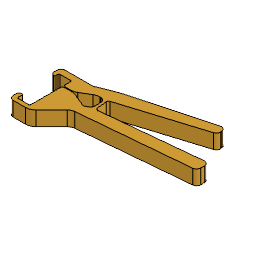
IOMOD-Puller (Autodesk Fusion 360 design; units mm, degrees)
Autodesk Fusion 360 part; units mm, degrees
note: some values were not read from the file. Set by a fixed rule: which sketch regions a step uses.
sketch "Sketch1" plane through (0, 0, 0) normal (0, 0, 1) x (1, 0, 0)
  line L0 (0, 5) -> (0, 2)
  line L1 (2, 0) -> (7.9289, 0)
  line L2 (11.4645, 1.4645) -> (18.976, 8.976)
  line L3 (21.4423, 10.1311) -> (73.1811, 14.8346)
  line L4 (75, 16.8264) -> (75, 18.7388)
  line L5 (72.7984, 20.7286) -> (26.4956, 16.038)
  line L6 (25.3999, 16.9322) -> (24.9151, 21.7179)
  line L7 (25.613, 22.7735) -> (63.4248, 34.5346)
  line L8 (64.8206, 36.6459) -> (64.76, 37.2443)
  line L9 (62.2441, 38.9723) -> (24.75, 28.75)
  line L10 (24.75, 28.75) -> (15.8665, 25.3333)
  line L11 (14.0716, 25) -> (2, 25)
  line L12 (0, 23) -> (0, 20.0001)
  line L13 (0, 20.0001) -> (1.5, 20.0001)
  line L14 (2, 20.5001) -> (2, 21.5)
  line L15 (2.5, 22) -> (7.5, 22)
  line L16 (8, 21.5) -> (8, 19)
  line L17 (9, 18) -> (11.6173, 18)
  line L18 (14.1909, 18.7132) -> (18.7957, 21.4777)
  line L19 (21.3693, 22.1909) -> (21.8547, 22.1909)
  line L20 (23.8445, 20.3925) -> (23.8704, 20.1372)
  line L21 (23.8704, 20.1372) -> (23.9618, 17.2187)
  line L22 (22.9342, 15.4078) -> (22.008, 14.8932)
  line L23 (8, 6.5218) -> (8, 2.5)
  line L24 (7.5, 2) -> (2.5, 2)
  line L25 (2, 2.5) -> (2, 4.5)
  line L26 (1.5, 5) -> (0, 5)
  arc A0 (23.8445, 20.3925) -> (21.8547, 22.1909) centre (21.8547, 20.1909) ccw
  arc A1 (73.1811, 14.8346) -> (75, 16.8264) centre (73, 16.8264) ccw
  arc A2 (75, 18.7388) -> (72.7984, 20.7286) centre (73, 18.7388) ccw
  arc A3 (63.4248, 34.5346) -> (64.8206, 36.6459) centre (62.8308, 36.4443) ccw
  arc A4 (64.76, 37.2443) -> (62.2441, 38.9723) centre (62.7702, 37.0427) ccw
  arc A5 (21.4423, 10.1311) -> (18.976, 8.976) centre (21.8044, 6.1475) ccw
  arc A6 (14.0716, 25) -> (15.8665, 25.3333) centre (14.0716, 30) ccw
  arc A7 (11.6173, 18) -> (14.1909, 18.7132) centre (11.6173, 23) ccw
  arc A8 (7.9289, 0) -> (11.4645, 1.4645) centre (7.9289, 5) ccw
  arc A9 (2, 25) -> (0, 23) centre (2, 23) ccw
  arc A10 (0, 2) -> (2, 0) centre (2, 2) ccw
  arc A11 (25.3999, 16.9322) -> (26.4956, 16.038) centre (26.3948, 17.0329) ccw
  arc A12 (25.613, 22.7735) -> (24.9151, 21.7179) centre (25.91, 21.8186) ccw
  arc A13 (21.3693, 22.1909) -> (18.7957, 21.4777) centre (21.3693, 17.1909) ccw
  arc A14 (8, 19) -> (9, 18) centre (9, 19) ccw
  arc A15 (8, 6.5247) -> (8, 6.5218) centre (9, 6.5218) ccw
  arc A16 (8, 21.5) -> (7.5, 22) centre (7.5, 21.5) ccw
  arc A17 (2.5, 22) -> (2, 21.5) centre (2.5, 21.5) ccw
  arc A18 (7.5, 2) -> (8, 2.5) centre (7.5, 2.5) ccw
  arc A19 (2, 2.5) -> (2.5, 2) centre (2.5, 2.5) ccw
  arc A20 (2, 4.5) -> (1.5, 5) centre (1.5, 4.5) ccw
  arc A21 (1.5, 20.0001) -> (2, 20.5001) centre (1.5, 20.5001) ccw
  line L27 (1, 5) -> (0, 4)
  line L28 (0.9999, 20.0001) -> (0, 21)
  arc A22 (22.9342, 15.4078) -> (23.9618, 17.2187) centre (21.9628, 17.1561) ccw
  line L29 (20.2644, 14.7966) -> (14.3954, 17.2531)
  line L30 (12.4649, 17.6408) -> (9.0149, 17.6408)
  line L31 (8.0149, 16.6422) -> (8, 6.5218)
  arc A23 (9.0149, 17.6408) -> (8.0149, 16.6422) centre (9.0149, 16.6408) ccw
  arc A24 (14.3954, 17.2531) -> (12.4649, 17.6408) centre (12.4649, 12.6408) ccw
  arc A25 (20.2644, 14.7966) -> (22.008, 14.8932) centre (21.0366, 16.6415) ccw
  point P0 (2, 5)
  dimension "d1" = 5
  dimension "d2" = 2
  dimension "d3" = 6
  dimension "d4" = 20
  dimension "d5" = 2
  dimension "d6" = 2
  dimension "d7" = 2
  dimension "d8" = 2
  dimension "d9" = 2
  dimension "d10" = 4
  dimension "d11" = 5
  dimension "d12" = 5
  dimension "d13" = 2
  dimension "d14" = 2
  dimension "d15" = 1
  dimension "d16" = 1
  dimension "d17" = 5
  dimension "d18" = 1
  dimension "d20" = 0.5
  dimension "d21" = 0.5
  dimension "d22" = 0.5
  dimension "d23" = 0.5
  dimension "d24" = 0.5
  dimension "d25" = 0.5
  dimension "d28" = 2
  dimension "d29" = 1
  dimension "d30" = 5
  dimension "d31" = 2
  constraint vertical L0
  constraint perpendicular L0 L1
  constraint perpendicular L1 L4
  constraint perpendicular L5 L6
  constraint perpendicular L5 L8
  constraint horizontal L11
  constraint perpendicular L11 L12
  constraint perpendicular L12 L13
  constraint perpendicular L13 L14
  constraint perpendicular L14 L15
  constraint perpendicular L15 L16
  constraint perpendicular L16 L17
  constraint parallel L17 L19
  constraint parallel L6 L20
  constraint vertical L23
  constraint perpendicular L23 L24
  constraint perpendicular L24 L25
  constraint perpendicular L0 L26
  constraint collinear L14 L25
  constraint collinear L16 L23
  constraint tangent L19 A0
  constraint tangent L20 A0
  constraint tangent L3 A1
  constraint tangent L4 A1
  constraint equal A0 A1
  constraint tangent L4 A2
  constraint tangent L5 A2
  constraint tangent L7 A3
  constraint tangent L8 A3
  constraint tangent L8 A4
  constraint tangent L9 A4
  constraint tangent L2 A5
  constraint tangent L3 A5
  constraint tangent L10 A6
  constraint tangent L11 A6
  constraint tangent L17 A7
  constraint tangent L18 A7
  constraint tangent L1 A8
  constraint tangent L2 A8
  constraint equal A7 A8
  constraint tangent L11 A9
  constraint tangent L12 A9
  constraint tangent L0 A10
  constraint tangent L1 A10
  constraint tangent L5 A11
  constraint tangent L6 A11
  constraint tangent L6 A12
  constraint tangent L7 A12
  constraint tangent L18 A13
  constraint tangent L19 A13
  constraint tangent L16 A14
  constraint tangent L17 A14
  constraint tangent L22 A15
  constraint tangent L23 A15
  constraint tangent L15 A16
  constraint tangent L16 A16
  constraint tangent L14 A17
  constraint tangent L15 A17
  constraint tangent L23 A18
  constraint tangent L24 A18
  constraint tangent L24 A19
  constraint tangent L25 A19
  constraint coincident P0 L25
  constraint coincident P0 L26
  constraint tangent L25 A20
  constraint tangent L26 A20
  constraint tangent L13 A21
  constraint tangent L14 A21
  constraint coincident L26 L27.start
  constraint coincident L0 L27.end
  constraint coincident L13 L28.start
  constraint coincident L12 L28.end
  constraint perpendicular L27 L28
  constraint tangent L21 A22
  constraint tangent L22 A22
  constraint parallel L11 L30
  constraint tangent L30 A23
  constraint tangent L31 A23
  constraint tangent L29 A24
  constraint tangent L30 A24
  constraint coincident L31 A15.start
  constraint tangent L29 A25
  constraint tangent L22 A25
  measures "d1" distance of L1 L26
  measures "d2" distance of L0.start P0
  measures "d3" distance of L23 L25
  measures "d4" distance of L15 L24
  measures "d5" distance of L1 L24
  measures "d6" radius of A0
  measures "d7" radius of A2
  measures "d8" radius of A3
  measures "d9" radius of A4
  measures "d10" radius of A5
  measures "d11" radius of A6
  measures "d12" radius of A7
  measures "d13" radius of A9
  measures "d14" radius of A10
  measures "d15" radius of A11
  measures "d16" radius of A12
  measures "d17" radius of A13
  measures "d18" radius of A14
  measures "d20" radius of A16
  measures "d21" radius of A17
  measures "d22" radius of A18
  measures "d23" radius of A19
  measures "d24" radius of A20
  measures "d25" radius of A21
  measures "d28" radius of A22
  measures "d29" radius of A23
  measures "d30" radius of A24
  measures "d31" radius of A25
extrude "Extrude1" add sketch "Sketch1" along normal blind 7 contours L0 L1 L2 L3 L4 L5 L6 L7 L8 L9 L10 L11 L12 L13 L14 L15 L16 L17 L18 L19 L20 L21 L22 L23 L24 L25 L26 A0 A1 A2 A3 A4 A5 A6 A7 A8 A9 A10 A11 A12 A13 A14 A15 A16 A17 A18 A19 A20 A21 L27 L28 A22 L29 L30 L31 A23 A24 A25
